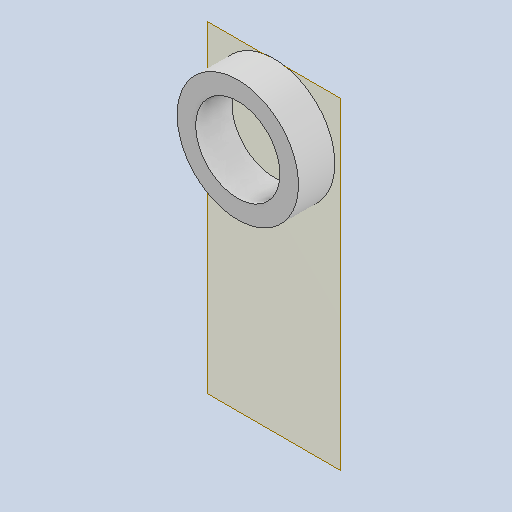
# Autodesk Inventor part: spacerA_V3
Saved by Autodesk Inventor 2023 (Build 270158000, 158)
## iProperties
Created: 2022-11-25
Part Number: spacerA_V3
Material: Generic
Document SubType Name: Modeling
Designer: shrey
Density: 1 g/cm^3
Appearance: Default
Author: shrey
Autodesk Inventor part; units mm, degrees
ref_plane "YZ Plane" through (0, 0, 0) normal (1, 0, 0) x (0, 1, 0)
ref_plane "XZ Plane" through (0, 0, 0) normal (0, 1, 0) x (-1, 0, 0)
ref_plane "XY Plane" through (0, 0, 0) normal (0, 0, 1) x (1, 0, 0)
ref_plane "Work Plane1" through (-7.7432, -45.9796, 22.0468) normal (0, 0, 1) x (1, 0, 0)
sketch "Sketch1" plane through (-7.7432, -45.9796, 22.0468) normal (0, 0, 1) x (1, 0, 0)
  spline S0 degree 3 number of poles 65 construction
  arc A0 (-1.7513, 49.5393) -> (-3.0984, 48.9393) centre (10.5928, 20.0161) ccw construction
  spline S1 degree 3 number of poles 65 construction
  arc A1 (-7.6198, 46.3277) -> (-8.8127, 45.4607) centre (10.5928, 20.0161) ccw construction
  spline S2 degree 3 number of poles 65 construction
  arc A2 (-12.6923, 41.9661) -> (-13.6789, 40.87) centre (10.5928, 20.0161) ccw construction
  spline S3 degree 3 number of poles 65 construction
  arc A3 (-16.7471, 36.6452) -> (-17.4843, 35.3679) centre (10.5928, 20.0161) ccw construction
  spline S4 degree 3 number of poles 65 construction
  arc A4 (-19.6071, 30.5975) -> (-20.0625, 29.1949) centre (10.5928, 20.0161) ccw construction
  spline S5 degree 3 number of poles 65 construction
  arc A5 (-21.1471, 24.0874) -> (-21.301, 22.6207) centre (10.5928, 20.0161) ccw construction
  spline S6 degree 3 number of poles 65 construction
  arc A6 (-21.3, 17.3993) -> (-21.1456, 15.9327) centre (10.5928, 20.0161) ccw construction
  spline S7 degree 3 number of poles 65 construction
  arc A7 (-20.059, 10.8256) -> (-19.603, 9.4231) centre (10.5928, 20.0161) ccw construction
  spline S8 degree 3 number of poles 65 construction
  arc A8 (-17.4784, 4.6536) -> (-16.7408, 3.3766) centre (10.5928, 20.0161) ccw construction
  spline S9 degree 3 number of poles 65 construction
  arc A9 (-13.6709, -0.8471) -> (-12.6839, -1.9428) centre (10.5928, 20.0161) ccw construction
  spline S10 degree 3 number of poles 65 construction
  arc A10 (-8.803, -5.4359) -> (-7.6098, -6.3025) centre (10.5928, 20.0161) ccw construction
  spline S11 degree 3 number of poles 65 construction
  arc A11 (-3.0874, -8.9123) -> (-1.7401, -9.5119) centre (10.5928, 20.0161) ccw construction
  spline S12 degree 3 number of poles 65 construction
  arc A12 (3.2261, -11.1244) -> (4.6687, -11.4307) centre (10.5928, 20.0161) ccw construction
  spline S13 degree 3 number of poles 65 construction
  arc A13 (9.8616, -11.9755) -> (11.3363, -11.9753) centre (10.5928, 20.0161) ccw construction
  spline S14 degree 3 number of poles 65 construction
  arc A14 (16.529, -11.4285) -> (17.9714, -11.1216) centre (10.5928, 20.0161) ccw construction
  spline S15 degree 3 number of poles 65 construction
  arc A15 (22.937, -9.5071) -> (24.2841, -8.9071) centre (10.5928, 20.0161) ccw construction
  spline S16 degree 3 number of poles 65 construction
  arc A16 (28.8054, -6.2955) -> (29.9983, -5.4284) centre (10.5928, 20.0161) ccw construction
  spline S17 degree 3 number of poles 65 construction
  arc A17 (33.8779, -1.9339) -> (34.8645, -0.8378) centre (10.5928, 20.0161) ccw construction
  spline S18 degree 3 number of poles 65 construction
  arc A18 (37.9328, 3.387) -> (38.6699, 4.6643) centre (10.5928, 20.0161) ccw construction
  spline S19 degree 3 number of poles 65 construction
  arc A19 (40.7927, 9.4347) -> (41.2482, 10.8373) centre (10.5928, 20.0161) ccw construction
  spline S20 degree 3 number of poles 65 construction
  arc A20 (42.3328, 15.9448) -> (42.4866, 17.4115) centre (10.5928, 20.0161) ccw construction
  spline S21 degree 3 number of poles 65 construction
  arc A21 (42.4856, 22.6329) -> (42.3312, 24.0995) centre (10.5928, 20.0161) ccw construction
  spline S22 degree 3 number of poles 65 construction
  arc A22 (41.2446, 29.2066) -> (40.7887, 30.6091) centre (10.5928, 20.0161) ccw construction
  spline S23 degree 3 number of poles 65 construction
  arc A23 (38.664, 35.3786) -> (37.9264, 36.6557) centre (10.5928, 20.0161) ccw construction
  spline S24 degree 3 number of poles 65 construction
  arc A24 (34.8565, 40.8793) -> (33.8695, 41.975) centre (10.5928, 20.0161) ccw construction
  spline S25 degree 3 number of poles 65 construction
  arc A25 (29.9886, 45.4681) -> (28.7954, 46.3347) centre (10.5928, 20.0161) ccw construction
  spline S26 degree 3 number of poles 65 construction
  arc A26 (24.273, 48.9445) -> (22.9257, 49.5441) centre (10.5928, 20.0161) ccw construction
  spline S27 degree 3 number of poles 65 construction
  arc A27 (17.9595, 51.1566) -> (16.517, 51.463) centre (10.5928, 20.0161) ccw construction
  spline S28 degree 3 number of poles 65 construction
  arc A28 (11.3241, 52.0077) -> (9.8493, 52.0075) centre (10.5928, 20.0161) ccw construction
  spline S29 degree 3 number of poles 65 construction
  arc A29 (4.6566, 51.4607) -> (3.2142, 51.1538) centre (10.5928, 20.0161) ccw construction
  circle A30 centre (10.5928, 20.0161) radius 6.16 construction
  line L0 (27.8335, 2.609) -> (17.5359, 14.0412) construction
  arc A31 (17.5359, 14.0412) -> (19.3648, 22.6538) centre (10.5928, 20.0161) ccw construction
  line L1 (19.3648, 22.6538) -> (33.4197, 28.9146) construction
  arc A32 (27.8335, 2.609) -> (33.4197, 28.9146) centre (10.5928, 20.0161) ccw construction
  line L2 (-0.6347, -1.7599) -> (7.0559, 11.5665) construction
  arc A33 (7.0559, 11.5665) -> (15.8121, 12.4885) centre (10.5928, 20.0161) ccw construction
  line L3 (15.8121, 12.4885) -> (26.1097, 1.0562) construction
  arc A34 (-0.6347, -1.7599) -> (26.1097, 1.0562) centre (10.5928, 20.0161) ccw construction
  line L4 (6.8765, 44.2326) -> (8.4877, 28.9309) construction
  arc A35 (8.4877, 28.9309) -> (1.9457, 23.0382) centre (10.5928, 20.0161) ccw construction
  line L5 (1.9457, 23.0382) -> (-13.1049, 26.2343) construction
  arc A36 (6.8765, 44.2326) -> (-13.1049, 26.2343) centre (10.5928, 20.0161) ccw construction
  line L6 (10.7949, 29.1739) -> (9.1837, 44.4755) construction
  arc A37 (32.4757, 31.0339) -> (9.1837, 44.4755) centre (10.5928, 20.0161) ccw construction
  line L7 (32.4757, 31.0339) -> (18.4208, 24.773) construction
  arc A38 (18.4208, 24.773) -> (10.7949, 29.1739) centre (10.5928, 20.0161) ccw construction
  line L8 (-13.5869, 23.965) -> (1.4638, 20.7688) construction
  arc A39 (1.4638, 20.7688) -> (5.0465, 12.7261) centre (10.5928, 20.0161) ccw construction
  line L9 (5.0465, 12.7261) -> (-2.6441, -0.6003) construction
  arc A40 (-13.5869, 23.965) -> (-2.6441, -0.6003) centre (10.5928, 20.0161) ccw construction
  circle A41 centre (10.5928, 20.0161) radius 5.86 construction
  circle A42 centre (10.5928, 20.0161) radius 3.86 construction
  circle A43 centre (10.5928, 20.0161) radius 6.36
  circle A44 centre (10.5928, 20.0161) radius 9.16
  point P0 (7.7432, 45.9796)
  dimension "d0" = 0.5
  constraints: 2 centre point, 1 coincident, 1 concentric
  measures "d0" radial gap between concentric circles of A41 A43
extrude "Extrusion1" add sketch "Sketch1" along normal blind 5.5
body "Solid1"
